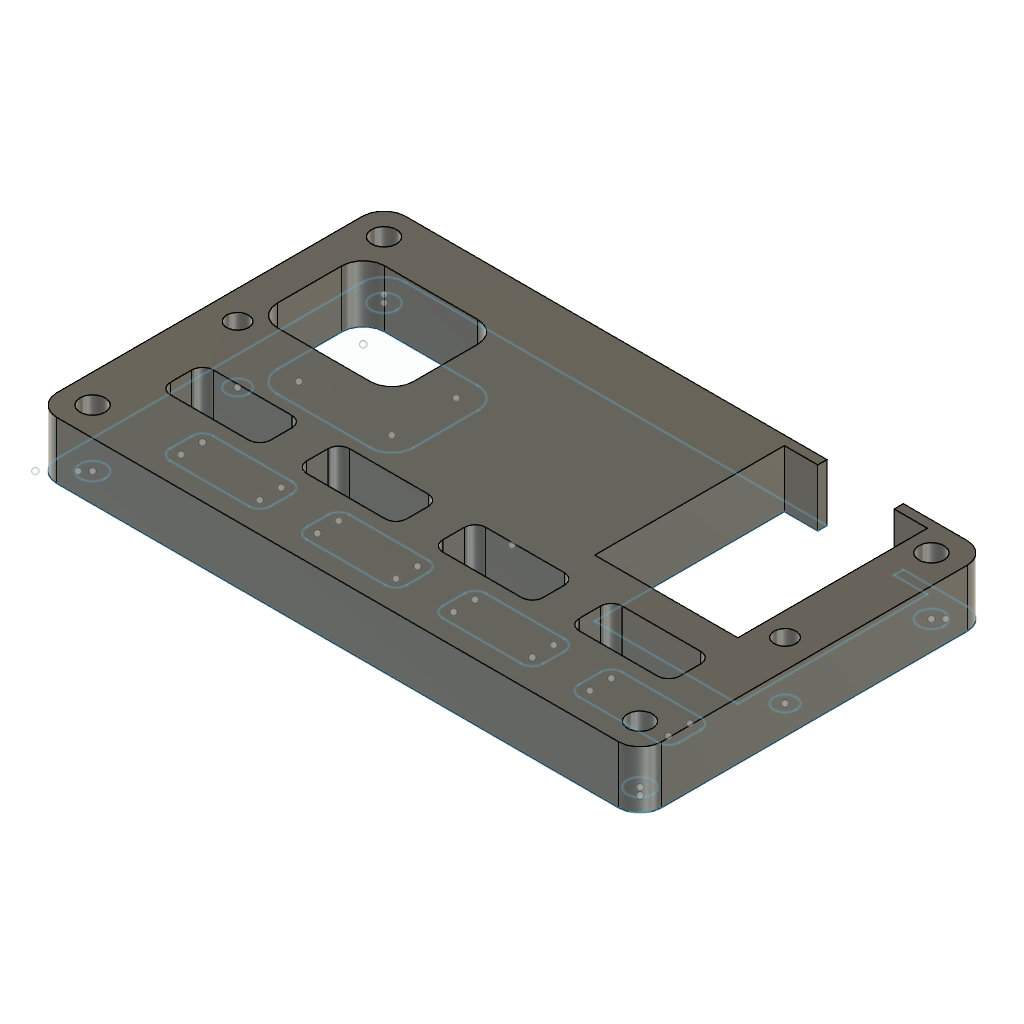
Hayai Lower midplate (Autodesk Fusion 360 design; units mm, degrees)
part number: 2026-09-20-19-27-11-121
Autodesk Fusion 360 part; units mm, degrees
sketch "Sketch1" plane through (0, 0, 0) normal (0, 0, 1) x (1, 0, 0)
  arc A0 (39.26, -24.3675) -> (42.26, -21.3675) centre (39.26, -21.3675) ccw
  circle A1 centre (38.26, -0.0995) radius 1.525
  circle A2 centre (-38.26, -20.3675) radius 1.75
  circle A3 centre (-38.26, 20.3675) radius 1.75
  line L0 (42.26, 21.3675) -> (42.26, -21.3675)
  arc A4 (-42.26, -21.3675) -> (-39.26, -24.3675) centre (-39.26, -21.3675) ccw
  line L1 (39.26, -24.3675) -> (-39.26, -24.3675)
  line L2 (-42.26, -21.3675) -> (-42.26, 21.3675)
  arc A5 (-39.26, 24.3675) -> (-42.26, 21.3675) centre (-39.26, 21.3675) ccw
  arc A6 (42.26, 21.3675) -> (39.26, 24.3675) centre (39.26, 21.3675) ccw
  circle A7 centre (38.26, 20.3675) radius 1.75
  circle A8 centre (-38.26, -0.0995) radius 1.525
  circle A9 centre (38.26, -20.3675) radius 1.75
  arc A10 (16.525, -9.1875) -> (15.025, -7.6875) centre (15.025, -9.1875) ccw
  arc A11 (-35.575, -12.1875) -> (-34.075, -13.6875) centre (-34.075, -12.1875) ccw
  line L3 (4.025, -7.6875) -> (15.025, -7.6875)
  arc A12 (-15.025, -7.6875) -> (-16.525, -9.1875) centre (-15.025, -9.1875) ccw
  line L4 (-16.525, -12.1875) -> (-16.525, -9.1875)
  line L5 (23.075, -13.6875) -> (34.075, -13.6875)
  line L6 (-15.025, -13.6875) -> (-4.025, -13.6875)
  arc A13 (21.575, -12.1875) -> (23.075, -13.6875) centre (23.075, -12.1875) ccw
  line L7 (-34.075, -7.6875) -> (-23.075, -7.6875)
  arc A14 (34.075, -13.6875) -> (35.575, -12.1875) centre (34.075, -12.1875) ccw
  line L8 (-34.075, -13.6875) -> (-23.075, -13.6875)
  line L9 (2.525, -12.1875) -> (2.525, -9.1875)
  arc A15 (35.575, -9.1875) -> (34.075, -7.6875) centre (34.075, -9.1875) ccw
  arc A16 (-2.525, -9.1875) -> (-4.025, -7.6875) centre (-4.025, -9.1875) ccw
  arc A17 (4.025, -7.6875) -> (2.525, -9.1875) centre (4.025, -9.1875) ccw
  line L10 (-35.575, -12.1875) -> (-35.575, -9.1875)
  line L11 (16.525, -12.1875) -> (16.525, -9.1875)
  arc A18 (-4.025, -13.6875) -> (-2.525, -12.1875) centre (-4.025, -12.1875) ccw
  line L12 (23.075, -7.6875) -> (34.075, -7.6875)
  arc A19 (-23.075, -13.6875) -> (-21.575, -12.1875) centre (-23.075, -12.1875) ccw
  line L13 (21.575, -12.1875) -> (21.575, -9.1875)
  line L14 (-15.025, -7.6875) -> (-4.025, -7.6875)
  line L15 (35.575, -12.1875) -> (35.575, -9.1875)
  arc A20 (2.525, -12.1875) -> (4.025, -13.6875) centre (4.025, -12.1875) ccw
  arc A21 (-16.525, -12.1875) -> (-15.025, -13.6875) centre (-15.025, -12.1875) ccw
  arc A22 (-21.575, -9.1875) -> (-23.075, -7.6875) centre (-23.075, -9.1875) ccw
  line L16 (-21.575, -12.1875) -> (-21.575, -9.1875)
  line L17 (-2.525, -12.1875) -> (-2.525, -9.1875)
  arc A23 (15.025, -13.6875) -> (16.525, -12.1875) centre (15.025, -12.1875) ccw
  arc A24 (-34.075, -7.6875) -> (-35.575, -9.1875) centre (-34.075, -9.1875) ccw
  line L18 (4.025, -13.6875) -> (15.025, -13.6875)
  arc A25 (23.075, -7.6875) -> (21.575, -9.1875) centre (23.075, -9.1875) ccw
  line L19 (-18.69, 4.8975) -> (-18.69, 13.8975)
  arc A26 (-18.69, 13.8975) -> (-21.69, 16.8975) centre (-21.69, 13.8975) ccw
  line L20 (-21.69, 16.8975) -> (-34.69, 16.8975)
  arc A27 (-34.69, 16.8975) -> (-37.69, 13.8975) centre (-34.69, 13.8975) ccw
  line L21 (-37.69, 4.8975) -> (-37.69, 13.8975)
  arc A28 (-37.69, 4.8975) -> (-34.69, 1.8975) centre (-34.69, 4.8975) ccw
  line L22 (-21.69, 1.8975) -> (-34.69, 1.8975)
  arc A29 (-21.69, 1.8975) -> (-18.69, 4.8975) centre (-21.69, 4.8975) ccw
  line L23 (35, -3.4325) -> (15, -3.4325)
  line L24 (19.67, 23.0675) -> (15, 23.0675)
  line L25 (30.33, 23.0675) -> (35, 23.0675)
  line L26 (15, -3.4325) -> (15, 23.0675)
  line L27 (35, 23.0675) -> (35, -3.4325)
  line L28 (19.67, 23.0675) -> (19.67, 24.3675)
  line L29 (30.33, 23.0675) -> (30.33, 24.3675)
  line L30 (39.26, 24.3675) -> (30.33, 24.3675)
  line L31 (19.67, 24.3675) -> (-39.26, 24.3675)
  point P0 (-42.26, -24.3675)
  dimension "d1" = 3.5
  dimension "d2" = 3.05
  dimension "d3" = 3.05
  dimension "d4" = 20.268
  dimension "d5" = 3
  dimension "d6" = 3
  dimension "d7" = 3
  dimension "d8" = 3
  dimension "d11" = 3.5
  dimension "d12" = 1.4142
  dimension "d13" = 4
  dimension "d14" = 10.68
  dimension "d15" = 6
  dimension "d16" = 14
  dimension "d17" = 1.5
  dimension "d18" = 1.5
  dimension "d19" = 1.5
  dimension "d20" = 1.5
  dimension "d21" = 1.5
  dimension "d22" = 1.5
  dimension "d23" = 1.5
  dimension "d24" = 1.5
  dimension "d25" = 1.5
  dimension "d26" = 1.5
  dimension "d27" = 1.5
  dimension "d28" = 1.5
  dimension "d29" = 1.5
  dimension "d30" = 1.5
  dimension "d31" = 1.5
  dimension "d32" = 1.5
  dimension "d33" = 6
  dimension "d34" = 6
  dimension "d35" = 6
  dimension "d36" = 10.68
  dimension "d37" = 10.68
  dimension "d38" = 10.68
  dimension "d40" = 6.685
  dimension "d41" = 5.05
  dimension "d42" = 5.05
  dimension "d43" = 5.05
  dimension "d44" = 4
  dimension "d45" = 4
  dimension "d46" = 4
  dimension "d47" = 1.4142
  dimension "d48" = 4
  dimension "d49" = 1.4142
  dimension "d50" = 20.268
  dimension "d51" = 14
  dimension "d52" = 14
  dimension "d53" = 14
  dimension "d54" = 6.685
  dimension "d55" = 3
  dimension "d56" = 3
  dimension "d57" = 3
  dimension "d58" = 3
  dimension "d59" = 19
  dimension "d60" = 15
  dimension "d61" = 4.57
  dimension "d63" = 26.5
  dimension "d64" = 26.5
  dimension "d65" = 20
  dimension "d66" = 10.66
  dimension "d67" = 1.3
  dimension "d68" = 1.3
  dimension "d69" = 4.67
  dimension "d70" = 4.67
  dimension "d71" = 7.26
  dimension "d78" = 3.5
  dimension "d79" = 3.5
  constraint vertical L0
  constraint horizontal L1
  constraint vertical L2
  constraint tangent L2 A5
  constraint tangent L0 A6
  constraint tangent A0 L0
  constraint tangent A0 L1
  constraint tangent A4 L1
  constraint tangent A4 L2
  constraint tangent A6 L30
  constraint tangent A5 L31
  measures "d1" diameter of A3
  measures "d2" diameter of A8
  measures "d3" diameter of A1
  measures "d4" distance of A2.centre A8.centre
  measures "d5" radius of A5
  measures "d6" radius of A6
  measures "d7" radius of A0
  measures "d8" radius of A4
  measures "d11" diameter of A9
  measures "d12" distance of A0.centre A9.centre
  measures "d13" distance of L1 A9.centre
  measures "d14" distance of L1 L8
  measures "d15" distance of L7 L8
  measures "d16" distance of L10 L16
  measures "d17" radius of A19
  measures "d18" radius of A22
  measures "d19" radius of A24
  measures "d20" radius of A11
  measures "d21" radius of A21
  measures "d22" radius of A12
  measures "d23" radius of A16
  measures "d24" radius of A18
  measures "d25" radius of A20
  measures "d26" radius of A17
  measures "d27" radius of A10
  measures "d28" radius of A23
  measures "d29" radius of A13
  measures "d30" radius of A25
  measures "d31" radius of A15
  measures "d32" radius of A14
  measures "d33" distance of L6 L14
  measures "d34" distance of L3 L18
  measures "d35" distance of L5 L12
  measures "d36" distance of L1 L6
  measures "d37" distance of L1 L5
  measures "d38" distance of L1 L18
  measures "d40" distance of L2 L10
  measures "d41" distance of L4 L16
  measures "d42" distance of L9 L17
  measures "d43" distance of L11 L13
  measures "d44" distance of A8.centre L2
  measures "d45" distance of A3.centre L2
  measures "d46" distance of A7.centre L0
  measures "d47" distance of A6.centre A7.centre
  measures "d48" distance of A1.centre L0
  measures "d49" distance of A5.centre A3.centre
  measures "d50" distance of A1.centre A9.centre
  measures "d51" distance of L4 L17
  measures "d52" distance of L9 L11
  measures "d53" distance of L13 L15
  measures "d54" distance of L0 L15
  measures "d55" radius of A28
  measures "d56" radius of A29
  measures "d57" radius of A26
  measures "d58" radius of A27
  measures "d59" distance of L19 L21
  measures "d60" distance of L20 L22
  measures "d61" distance of L2 L21
  measures "d63" distance of L23 L24
  measures "d64" distance of L23 L25
  measures "d65" distance of L26 L27
  measures "d66" distance of L28 L29
  measures "d67" distance of L24.start L28.end
  measures "d68" distance of L29.end L25.start
  measures "d69" distance of L24.end L28
  measures "d70" distance of L25.end L29
  measures "d71" distance of L0 L27
  measures "d78" diameter of A2
  measures "d79" diameter of A7
extrude "Extrude1" add sketch "Sketch1" along normal blind 3
extrude "Extrude2" add 1 faces at (0.0405, 9.7541, 3) along direction (0, 0, 1) blind 4
extrude "Extrude4" add 1 faces at (0.0405, 9.7541, 7) along direction (0, 0, 1) blind 1
